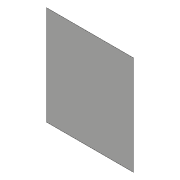
# Autodesk Inventor part: plinthScreen
Saved by Autodesk Inventor 2017 (Build 210142000, 142)
## iProperties
Created: 2016-11-30
Part Number: plinthScreen
Material: Generic
Document SubType Name: Modeling
Designer: krosie
Density: 1 g/cm^3
Appearance: Default
Author: krosie
Autodesk Inventor part; units mm, degrees
ref_plane "YZ Plane" through (0, 0, 0) normal (1, 0, 0) x (0, 1, 0)
ref_plane "XZ Plane" through (0, 0, 0) normal (0, 1, 0) x (-1, 0, 0)
ref_plane "XY Plane" through (0, 0, 0) normal (0, 0, 1) x (1, 0, 0)
sketch "Sketch3" plane through (0, 0, 0) normal (0, 1, 0) x (-1, 0, 0)
  line L0 (-368.3, 419.1) -> (368.3, 419.1)
  line L1 (368.3, 419.1) -> (368.3, -419.1)
  line L2 (368.3, -419.1) -> (-368.3, -419.1)
  line L3 (-368.3, -419.1) -> (-368.3, 419.1)
  line L4 (-368.3, 419.1) -> (368.3, -419.1) construction
  line L5 (368.3, 419.1) -> (-368.3, -419.1) construction
  point P0 (0, 0)
  dimension "d8" = 736.6
  dimension "d9" = 838.2
  constraints: 12 end point, 2 midpoint, 2 parallel, 1 horizontal, 1 perpendicular
  measures "d8" distance of L1.end L2.end
  measures "d9" distance of L0.end L1.end
extrude "Extrusion1" add sketch "Sketch3" along normal blind 0.71
body "Solid2"
